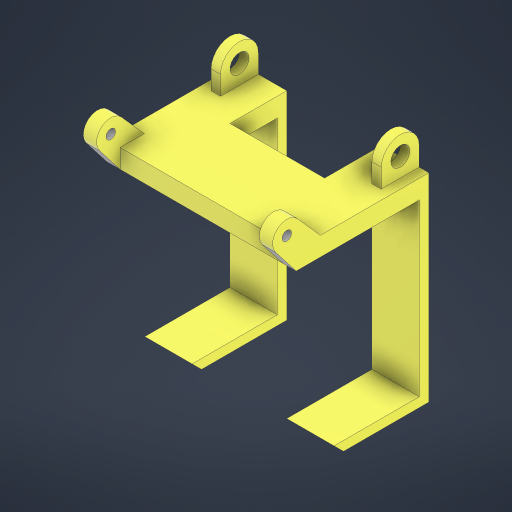
# Autodesk Inventor part: FP V2 Claw
Saved by Autodesk Inventor 2023.6 (Build 276521000, 521)
## iProperties
Created: 2026-02-19
Part Number: FP V2 Claw
Material: Generic
Document SubType Name: Modeling
Designer: user
Density: 1 g/cm^3
Appearance: Default
Author: user
Autodesk Inventor part; units mm, degrees
sketch "Sketch1" plane through (0, 0, 0) normal (0, 0, 1) x (1, 0, 0)
  line L0 (0, 0) -> (50, 0)
  line L1 (0, 0) -> (-50, 0)
  line L2 (-50, 0) -> (-50, 5)
  line L3 (-50, 5) -> (50, 5)
  line L4 (50, 5) -> (50, 0)
  dimension "d0" = 50
  dimension "d1" = 50
  dimension "d2" = 5
  constraints: 10 end point, 2 horizontal, 2 perpendicular, 1 vertical
  measures "d0" distance of L0.start L0.end
  measures "d1" distance of L0.start L1.end
  measures "d2" distance of L1.end L2.end
extrude "Extrusion1" add sketch "Sketch1" against normal blind 40
sketch "Sketch2" plane through (-50, 0, 0) normal (0, -1, 0) x (1, 0, 0)
  line L0 (0, 0) -> (0, -40) projected
  line L1 (0, 0) -> (0, -40) projected
  line L2 (100, -40) -> (0, -40) projected
  line L3 (0, 0) -> (100, 0) projected
  line L4 (0, -40) -> (100, -40) projected
  line L5 (100, 0) -> (0, 0) projected
  line L6 (100, 0) -> (100, -40) projected
  line L7 (100, 0) -> (100, -40) projected
  point P0 (50, 0)
extrude "Extrusion2" add sketch "Sketch2" along normal blind 100
shell "Shell1" thickness 5 removed faces 3 at (-16.6667, -30, 0) at (50, -65, -13.3333) at (-50, -30, -13.3333)
sketch "Sketch3" plane through (0, 0, 0) normal (0, 0, 1) x (1, 0, 0)
  line L0 (50, -95) -> (-50, -95) projected
  line L1 (-50, -95) -> (-50, -100) projected
  line L2 (50, -100) -> (-50, -100) projected
  line L3 (50, -100) -> (50, -95) projected
  point P0 (0, 0)
extrude "Extrusion3" add sketch "Sketch3" along normal blind 30
sketch "Sketch4" plane through (50, 5, 0) normal (1, 0, 0) x (0, 0, -1)
  line L0 (-30, -105) -> (-30, -100) projected
  line L1 (-30, -100) -> (-25, -105)
  line L2 (40, -105) -> (-30, -105) projected
  point P0 (0, -5)
  dimension "d10" = 45
  constraints: 2 end point, 1 point on line
  measures "d10" angle of L2 L1
extrude "Extrusion4" cut sketch "Sketch4" against normal through all
sketch "Sketch5" plane through (-50, -95, -35) normal (0, 1, 0) x (1, 0, 0)
  line L0 (100, -60) -> (0, -60) projected
  line L1 (0, 5) -> (0, -60) projected
  line L2 (0, 5) -> (100, 5) projected
  line L3 (100, 5) -> (100, -60) projected
  line L4 (0, -60) -> (0, -65) projected
  line L5 (100, -60) -> (0, -60) projected
  line L6 (100, -65) -> (100, -60) projected
  line L7 (100, -65) -> (0, -65) projected
  line L8 (25, -5) -> (75, -5)
  line L9 (75, -5) -> (75, -65)
  line L10 (75, -65) -> (25, -65)
  line L11 (25, -65) -> (25, -5)
  line L12 (25, -5) -> (75, -65) construction
  line L13 (75, -5) -> (25, -65) construction
  point P0 (50, -35)
  dimension "d13" = 25
  constraints: 12 end point, 2 midpoint, 2 parallel, 1 horizontal, 1 perpendicular, 1 point on line
  measures "d13" distance between parallel lines of L3 L9
extrude "Extrusion5" cut sketch "Sketch5" against normal blind 10 contours L9 L7 L11 L0 | L0 L11 L8 L9
sketch "Sketch6" plane through (0, 0, 0) normal (0, 0, 1) x (1, 0, 0)
  line L0 (-50, 0) -> (50, 0) projected
  line L1 (50, 0) -> (50, 5) projected
  line L2 (50, 5) -> (-50, 5) projected
  line L3 (-50, 5) -> (-50, 0) projected
  point P0 (0, 0)
extrude "Extrusion6" add sketch "Sketch6" along normal up to surface (30 mm away)
sketch "Sketch7" plane through (-50, 0, -35) normal (0, -1, 0) x (1, 0, 0)
  line L0 (0, 0) -> (0, 65) projected
  line L1 (0, 0) -> (100, 0) projected
  line L2 (100, 65) -> (100, 0) projected
  line L3 (100, 65) -> (0, 65) projected
  point P0 (50, 35)
extrude "Extrusion7" add sketch "Sketch7" along normal blind 5
sketch "Sketch8" plane through (-50, -100, -40) normal (-1, 0, 0) x (0, 0, 1)
  line L0 (0, 105) -> (70, 105) projected
  line L1 (70, 105) -> (75, 113.6603)
  line L2 (70, 105) -> (70, 95) projected
  line L3 (70, 95) -> (87.3602, 125.0687)
  circle A0 centre (75, 113.6603) radius 5
  line L4 (70.6699, 116.1603) -> (64.2265, 105)
  circle A1 centre (75, 113.6603) radius 7.5
  line L5 (69.3926, 118.6409) -> (57.2762, 105)
  line L6 (0, 105) -> (70, 105) projected
  line L7 (70, 105) -> (70, 95) projected
  line L8 (80.9226, 109.0589) -> (70, 95)
  point P0 (40, 100)
  point P1 (82.1252, 116.0015)
  point P2 (67.8748, 111.319)
  point P3 (76.535, 106.319)
  dimension "d20" = 120
  dimension "d21" = 10
  dimension "d22" = 15
  constraints: 10 end point, 2 coincident, 2 parallel, 2 point on circle, 2 point on line, 2 tangent, 1 centre point, 5 other
  measures "d20" angle of L0 L1
  measures "d21" distance of L0.end L1.end
  measures "d22" diameter of A1
extrude "Extrusion8" add sketch "Sketch8" against normal blind 7 contours L5 A1 L4 L0 | L4 A1 L1 L0 | A1 L3 A0 L4 | L1 A1 L3 L2 | L4 A0 L1 A1 | A1 L3 | L1 A0 L3 A1 | L3 A1 L8
ref_plane "Work Plane1" through (0, -100, -40) normal (-1, 0, 0) x (0, 0, 1)
mirror "Mirror1" about plane through (0, -100, -40) normal (-1, 0, 0) of "Extrusion8"
sketch "Sketch9" plane through (0, 0, -40) normal (0, 0, -1) x (-1, 0, 0)
  line L0 (-25, -100) -> (25, -100) projected
  line L1 (-25, -100) -> (-25, 10)
  line L2 (-25, 10) -> (25, 10)
  line L3 (25, 10) -> (25, -100)
  point P0 (0, 0)
  dimension "d25" = 110
  constraints: 6 end point, 2 perpendicular, 1 vertical
  measures "d25" distance of L0.start L1.end
extrude "Extrusion9" cut sketch "Sketch9" against normal blind 30
sketch "Sketch10" plane through (-50, -100, -40) normal (-1, 0, 0) x (0, 0, 1)
  line L0 (65, 0) -> (70, 5) projected
  line L1 (70, 5) -> (50, 5)
  line L2 (70, 5) -> (5, 5) projected
  line L3 (50, 5) -> (45, 0)
  line L4 (0, 0) -> (65, 0) projected
  line L5 (65, 0) -> (70, 5) projected
  point P0 (40, 100)
  dimension "d28" = 20
  constraints: 4 end point, 2 point on line, 1 parallel
  measures "d28" distance of L0.end L1.end
extrude "Extrusion10" cut sketch "Sketch10" against normal through all
sketch "Sketch11" plane through (-50, -100, -40) normal (-1, 0, 0) x (0, 0, 1)
  circle A0 centre (10, 115) radius 10
  circle A1 centre (10, 115) radius 5
  line L0 (0, 105) -> (57.2762, 105) projected
  line L1 (0, 105) -> (0, 115)
  line L2 (0, 105) -> (57.2762, 105) projected
  line L3 (20, 115) -> (20, 105)
  point P0 (40, 100)
  point P1 (64.2265, 105)
  dimension "d31" = 20
  dimension "d32" = 10
  dimension "d33" = 10
  constraints: 4 end point, 3 vertical, 1 centre point, 1 coincident, 1 horizontal, 1 perpendicular, 1 point on line, 3 other
  measures "d32" diameter of A1
  measures "d33" distance of L0.start L1.end
extrude "Extrusion11" add sketch "Sketch11" against normal blind 5
ref_plane "Work Plane2" through (0, -100, -40) normal (1, 0, 0) x (0, 0, -1)
mirror "Mirror2" about plane through (0, -100, -40) normal (1, 0, 0) of "Extrusion11"
sketch "Sketch12" plane through (-45, -100, -40) normal (1, 0, 0) x (0, 0, -1)
  arc A0 (0, 115) -> (-20, 115) centre (-10, 115) ccw projected
  line L0 (-20, 115) -> (-20, 105) projected
  line L1 (0, 105) -> (-20, 105) projected
  line L2 (0, 105) -> (0, 115) projected
  circle A1 centre (-10, 115) radius 5 projected
  point P0 (-40, 100)
extrude "Extrusion12" add sketch "Sketch12" along normal blind 5
extrude "Extrusion13" cut sketch "Sketch12" against normal blind 5 contours L2 L1 L0 A0 | A1
ref_plane "Work Plane3" through (0, -95, -35) normal (1, 0, 0) x (0, 0, -1)
mirror "Mirror3" about plane through (0, -95, -35) normal (1, 0, 0) of "Extrusion11", "Extrusion12", "Extrusion13"
sketch "Sketch13" plane through (-50, -100, -40) normal (-1, 0, 0) x (0, 0, 1)
  circle A0 centre (75, 113.6603) radius 5 projected
  circle A1 centre (75, 113.6603) radius 2.5
  circle A2 centre (75, 113.6603) radius 5
  point P0 (40, 100)
  dimension "d40" = 5
  constraints: 2 centre point, 2 coincident, 1 concentric
  measures "d40" diameter of A1
extrude "Extrusion14" add sketch "Sketch13" against normal blind 7
mirror "Mirror4" about plane through (0, -95, -35) normal (1, 0, 0) of "Extrusion14"
body "Solid1"
